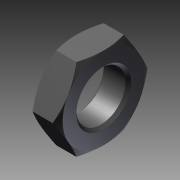
# Autodesk Inventor part: V-12-16
Saved by Autodesk Inventor 2011 SP1 (Build 150282100, 282)
## iProperties
Created: 2018-01-08
Part Number: V-12-16
Catalog Web Link: www.cadenas.de
Description: Mod. V-Nose Nut
Vendor: CAMOZZI
Document SubType Name: Modeling
Designer: psAdmin
Manufacturer: CAMOZZI
Mass: 2.63116 g
Surface Area: 16.1143 cm^2
Volume: 2.63116 cm^3
Density: 1 g/cm^3
Category: PARTsolutions
Company: CAMOZZI
Title: V-12-16
Author: Cadenas PARTsolutions
Comments: Nose Nut
PSOL_IDENT_0: {$CADENAS_DATA\23d-libs\camozzi\movimento\cilindri_a_norma_e_cilindri_standard\minicilindri_serie_16
PSOL_IDENT_1: _24_25\accessori\ghiera_mod_v.prj},147 {VTYP=3D},{NB=V-12-16},{LINA=V-12-16},{NN=Mod. V},{DATE=27.07
PSOL_IDENT_2: .2017 08:45:31},{GEOMDATE=16.03.2006},{VERSION=},{LINEID=20},{LINESUBID=-1},{WBVAR=}  {NB=V-12-16},{
PSOL_IDENT_3: LINA=V-12-16},{KT=DUMMY},{IDNR=},{MOD=V-12-16},{PHY=12 - 16},{D=M16x1.5},{M=8},{SW=24},{DNDM=16.0},{
PSOL_IDENT_4: DKDM=14.37619},{P=1.50},{INFO=Infotext}
NN: Mod. V
NT: Nose Nut
NB: V-12-16
NBSYN: $MOD.
LINA: V-12-16
MOD: V-12-16
PHY: 12 - 16
D: M16x1.5
M: 8
SW: 24
INFO: Infotext
SUPPLIER: CAMOZZI
ARTICLENO: V-12-16
BOMINFO: V-12-16
CREATOR: CADENAS GmbH
Autodesk Inventor part; units mm, degrees
sketch "Skizze_1" plane through (0, 0, 0) normal (0, 0, 1) x (1, 0, 0)
  line L0 (8, 0) -> (0, 0)
  line L1 (0, 0) -> (0, 12)
  line L2 (0, 12) -> (1.3856, 14.4)
  line L3 (1.3856, 14.4) -> (6.6144, 14.4)
  line L4 (6.6144, 14.4) -> (8, 12)
  line L5 (8, 12) -> (8, 0)
  line L6 (8, 0) -> (0, 0)
  constraints: 14 end point
revolve "Revolution1" add sketch "Skizze_1" angle 360 about axis through (8, 0, 0) along (1, 0, 0)
sketch "Skizze_2_ALT_Drilling_1" plane through (0, 0, 0) normal (0, 0, 1) x (1, 0, 0)
  line L0 (8, 0) -> (0, 0)
  line L1 (0, 0) -> (0, 8)
  line L2 (0, 8) -> (0.8119, 7.1881)
  line L3 (0.8119, 7.1881) -> (7.1881, 7.1881)
  line L4 (7.1881, 7.1881) -> (8, 8)
  line L5 (8, 8) -> (8, 0)
  line L6 (8, 0) -> (0, 0)
  constraints: 14 end point
revolve "Revolution2" cut sketch "Skizze_2_ALT_Drilling_1" angle 360 about axis through (8, 0, 0) along (1, 0, 0)
sketch "Skizze_3" plane through (0, 0, 0) normal (1, 0, 0) x (0, 1, 0)
  line L0 (-24, 24) -> (-24, -24)
  line L1 (-24, -24) -> (24, -24)
  line L2 (24, -24) -> (24, 24)
  line L3 (24, 24) -> (-24, 24)
  line L4 (-6.9282, 12) -> (-13.8564, 0)
  line L5 (-13.8564, 0) -> (-6.9282, -12)
  line L6 (-6.9282, -12) -> (6.9282, -12)
  line L7 (6.9282, -12) -> (13.8564, 0)
  line L8 (13.8564, 0) -> (6.9282, 12)
  line L9 (6.9282, 12) -> (-6.9282, 12)
  constraints: 20 end point
extrude "Extrusion1" cut sketch "Skizze_3" along normal blind 8
ref_plane "GIE1_XY" through (0, 0, 0) normal (1, 0, 0) x (0, 0, -1)
ref_plane "GIE1_YZ" through (0, 0, 0) normal (0, 0, -1) x (0, 1, 0)
ref_plane "GIE1_ZX" through (0, 0, 0) normal (0, 1, 0) x (1, 0, 0)
body "Solid1"
